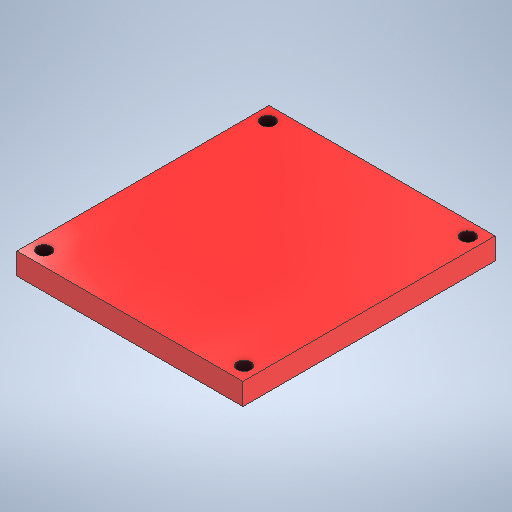
# Autodesk Inventor part: L298N module base
Saved by Autodesk Inventor 2025.3 (Build 293356000, 356)
## iProperties
Created: 2025-12-05
Part Number: L298N module base
Material: Generic
Document SubType Name: Modeling
Designer: maxim
Density: 1 g/cm^3
Appearance: 12in Running - Burgundy
Author: maxim
Autodesk Inventor part; units mm, degrees
ref_plane "YZ Plane" through (0, 0, 0) normal (1, 0, 0) x (0, 1, 0)
ref_plane "XZ Plane" through (0, 0, 0) normal (0, 1, 0) x (-1, 0, 0)
ref_plane "XY Plane" through (0, 0, 0) normal (0, 0, 1) x (1, 0, 0)
sketch "Sketch1" plane through (0, 0, 0) normal (0, 1, 0) x (-1, 0, 0)
  line L0 (0, 0) -> (-52, 0)
  line L1 (-52, 0) -> (-52, -58)
  line L2 (-52, -58) -> (0, -58)
  line L3 (0, -58) -> (0, 0)
  line L4 (-49, -54.75) -> (-49, -3.25) construction
  line L5 (-49, -54.75) -> (-3, -54.75) construction
  point P0 (-3, -3.25)
  point P1 (-49, -29)
  point P2 (-52, -29)
  point P3 (-26, -54.75)
  point P4 (-26, -58)
  dimension "d0" = 52
  dimension "d1" = 58
  dimension "d15" = 51.5
  dimension "d16" = 46
  constraints: 12 end point, 4 midpoint, 3 horizontal alignment, 3 vertical alignment, 2 horizontal, 2 parallel, 2 perpendicular
  measures "d0" distance of L2.end L1.end
  measures "d1" distance of L0.end L1.end
  measures "d15" distance of L4.end L4.start
  measures "d16" distance of L4.start L5.end
extrude "Extrusion1" add sketch "Sketch1" along normal blind 5
hole "Hole1" at (3, 0, -54.75) at (3, 0, -3.25) at (49, 0, -3.25) at (49, 0, -54.75) direction (0, 1, 0) diameter 3.2 end through all
body "Solid1"
